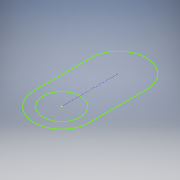
# Autodesk Inventor part: Extruder Clamp
Saved by Autodesk Inventor 2018 (Build 220112000, 112)
## iProperties
Created: 2018-05-13
Part Number: Extruder Clamp
Material: Generic
Document SubType Name: Modeling
Designer: Jasper
Density: 1 g/cm^3
Appearance: Default
Author: Jasper
Autodesk Inventor part; units mm, degrees
ref_plane "YZ Plane" through (0, 0, 0) normal (1, 0, 0) x (0, 1, 0)
ref_plane "XZ Plane" through (0, 0, 0) normal (0, 1, 0) x (-1, 0, 0)
ref_plane "XY Plane" through (0, 0, 0) normal (0, 0, 1) x (1, 0, 0)
sketch "Sketch1" plane through (0, 0, 0) normal (0, 0, 1) x (1, 0, 0)
  circle A0 centre (0, 0) radius 2.7
  line L0 (0, 0) -> (0, 13) construction
  line L1 (-6.7, 0) -> (-6.7, 13)
  line L2 (6.7, 13) -> (6.7, 0)
  arc A1 (-6.7, 0) -> (6.7, 0) centre (0, 0) ccw
  arc A2 (6.7, 13) -> (-6.7, 13) centre (0, 13) ccw
  circle A3 centre (0, 0) radius 2.5 construction
  line L3 (-35, 15.2) -> (0, 15.2) construction
  line L4 (-35, 10.7) -> (0, 10.7)
  line L5 (0, 19.7) -> (-35, 19.7)
  arc A4 (-35, 19.7) -> (-35, 10.7) centre (-35, 15.2) ccw
  arc A5 (0, 10.7) -> (0, 19.7) centre (0, 15.2) ccw
  line L6 (0, 13) -> (0, 19.7) construction
  circle A6 centre (3, 15.5) radius 1.5 construction
  circle A7 centre (3, 15.5) radius 5
  point P0 (0, 6.5)
  point P1 (-17.5, 15.2)
  dimension "d2" = 0.2
  dimension "d3" = 4
  dimension "d5" = 13
  dimension "d10" = 9
  dimension "d11" = 35
  dimension "d12" = 10
  constraints: 18 end point, 9 point on circle, 8 tangent, 6 centre point, 2 coincident, 2 midpoint, 2 parallel, 1 horizontal, 1 vertical
  measures "d2" radial gap between concentric circles of A0 A3
  measures "d3" radial gap between concentric circles of A1 A0
  measures "d5" distance of L0.start L0.end
  measures "d10" distance between parallel lines of L4 L5
  measures "d11" distance of L3.start L3.end
  measures "d12" diameter of A7
extrude "Extrusion1" add sketch "Sketch1" along normal blind 13
sketch "Sketch8" plane through (0, 0, 13) normal (0, 0, 1) x (1, 0, 0)
  line L0 (0, 2.7) -> (-16.9826, 2.7)
  line L1 (-16.9826, -2.7) -> (0, -2.7)
  arc A0 (0, -2.7) -> (0, 2.7) centre (0, 0) ccw
  arc A1 (-16.9826, 2.7) -> (-16.9826, -2.7) centre (-16.9826, 0) ccw
  circle A2 centre (0, 0) radius 2.7 construction
  line L2 (-16.9826, 0) -> (0, 0) construction
  point P0 (-3.3627, 0)
  dimension "d25" = 16.9826
  constraints: 6 end point, 5 tangent, 4 point on circle, 2 centre point, 1 horizontal, 1 parallel
  measures "d25" distance of L2.start L2.end
extrude "Extrusion6" cut sketch "Sketch8" against normal through all
sketch "Sketch9" plane through (0, 0, 13) normal (0, 0, 1) x (1, 0, 0)
  arc A0 (0, -2.7) -> (0, 2.7) centre (0, 0) ccw construction
  arc A1 (-6.1319, -2.7) -> (6.7, 0) centre (0, 0) ccw construction
  line L0 (0, 0) -> (0, 13) construction
  line L1 (6.7, 0) -> (6.7, 13)
  line L2 (-6.7, 13) -> (-6.7, 0)
  arc A2 (-6.7, 0) -> (6.7, 0) centre (0, 0) ccw
  arc A3 (6.7, 13) -> (-6.7, 13) centre (0, 13) ccw construction
  line L3 (0, 19.7) -> (-35, 19.7) projected
  line L4 (-6.7, 13) -> (6.7, 13)
  point P0 (0, 6.5)
  constraints: 10 end point, 6 tangent, 4 point on circle, 2 centre point, 1 midpoint, 1 parallel, 1 perpendicular, 1 vertical
extrude "Extrusion7" add sketch "Sketch9" against normal blind 1
ref_plane "Work Plane1" through (0, 0, 6.5) normal (0, 0, 1) x (1, 0, 0)
mirror "Mirror3" about plane through (0, 0, 6.5) normal (0, 0, 1) of "Extrusion7"
sketch "Sketch2" plane through (-35, 19.7, 0) normal (0, 1, 0) x (1, 0, 0)
  circle A0 centre (12, -3) radius 1.6 construction
  line L0 (52.5, -6.5) -> (-14, -6.5) construction
  line L1 (9.5, -3) -> (14.5, -3) construction
  line L2 (9.5, -4.75) -> (14.5, -4.75)
  line L3 (14.5, -1.25) -> (9.5, -1.25)
  arc A1 (9.5, -1.25) -> (9.5, -4.75) centre (9.5, -3) ccw
  arc A2 (14.5, -4.75) -> (14.5, -1.25) centre (14.5, -3) ccw
  point P0 (35, 0)
  dimension "d6" = 3.5
  dimension "d7" = 5
  constraints: 8 end point, 4 point on circle, 4 tangent, 2 centre point, 1 horizontal, 1 midpoint, 1 parallel
  measures "d6" distance between parallel lines of L2 L3
  measures "d7" distance of L1.start L1.end
extrude "Extrusion2" cut sketch "Sketch2" against normal through all
ref_plane "Work Plane2" through (0, 0, 0) normal (1, 0, 0) x (0, 0, -1)
sketch "Sketch4" plane through (0, 0, 0) normal (1, 0, 0) x (0, 0, -1)
  line L0 (-4, -7.79) -> (-4, 7.79) construction
  line L1 (-8.79, -8) -> (-4.21, -8) construction
  line L2 (-9, -7.79) -> (-9, 7.79) construction
  line L3 (-8.79, 8) -> (-4.21, 8) construction
  line L4 (-4.21, 8) -> (-4, 8) construction
  line L5 (-4, 8) -> (-4, 7.79) construction
  line L6 (-9, -7.79) -> (-9, -8) construction
  line L7 (-9, -8) -> (-8.79, -8) construction
  line L8 (-4, 8) -> (-9, -8) construction
  line L9 (-10, -9) -> (-3, -9)
  line L10 (-3, -9) -> (-3, 9)
  line L11 (-3, 9) -> (-10, 9)
  line L12 (-10, 9) -> (-10, -9)
  line L13 (0, 0) -> (-13, 0) projected
  line L14 (-10, -9) -> (-3, 9) construction
  line L15 (-3, -9) -> (-10, 9) construction
  line L16 (-3, 0) -> (-10, 0)
  point P0 (-6.5, 0)
  dimension "d15" = 1
  dimension "d16" = 1
  constraints: 28 end point, 5 midpoint, 4 horizontal, 3 perpendicular, 2 parallel, 2 point on line, 1 vertical, 4 other
  measures "d15" distance between parallel lines of L0 L10
  measures "d16" distance between parallel lines of L11 L3
revolve "Revolution1" cut sketch "Sketch4" angle 360 about axis through (0, 0, 0) along (0, 0, 1) contours L12 L13 L10 L9
sketch "Sketch5" plane through (0, 0, 13) normal (0, 0, 1) x (1, 0, 0)
  arc A0 (6.7, 12.137) -> (0.2781, 19.6942) centre (3, 15.5) ccw construction
  circle A1 centre (3, 15.5) radius 1.75
  point P0 (0, 0)
  dimension "d18" = 3.5
  constraints: 1 centre point, 1 coincident
  measures "d18" diameter of A1
extrude "Extrusion3" cut sketch "Sketch5" against normal through all
sketch "Sketch7" plane through (0, 0, 3) normal (0, 0, 1) x (0.9785721, 0.2059046, 0)
  line L0 (0, 0) -> (0, 9) construction
  arc A0 (7.7937, 4.5008) -> (-5.3191, 7.26) centre (0, 0) ccw construction
  line L1 (-6.7, -9) -> (6.7, -9)
  line L2 (6.7, -9) -> (6.7, 9)
  line L3 (6.7, 9) -> (-6.7, 9)
  line L4 (-6.7, 9) -> (-6.7, -9)
  line L5 (-6.7, -9) -> (6.7, 9) construction
  line L6 (6.7, -9) -> (-6.7, 9) construction
  line L7 (7.7937, 4.5008) -> (6.5564, -1.3796) construction
  line L8 (-6.7, -9) -> (0, -9)
  line L9 (0, -9) -> (0, 9)
  line L10 (0, 9) -> (-6.7, 9)
  line L11 (-6.7, 9) -> (-6.7, -9)
  constraints: 22 end point, 4 parallel, 2 horizontal, 2 midpoint, 2 perpendicular, 1 point on circle, 1 tangent, 1 vertical, 1 other
extrude "Extrusion5" cut sketch "Sketch7" along normal up to surface (7 mm away) contours L4 L3 L9 L1
mirror "Mirror4" about plane through (0, 0, 6.5) normal (0, 0, 1) of "Extrusion2"
body "Solid1"
